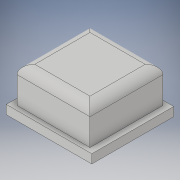
# Autodesk Inventor part: BUTTON2
Saved by Autodesk Inventor 2019 (Build 230136000, 136)
## iProperties
Created: 2018-12-20
Part Number: BUTTON2
Material: Типовые
Document SubType Name: Modeling
Designer: aldanstar
Density: 1 g/cm^3
Appearance: По умолчанию
Author: aldanstar
Autodesk Inventor part; units mm, degrees
ref_plane "YZ Plane" through (0, 0, 0) normal (1, 0, 0) x (0, 1, 0)
ref_plane "XZ Plane" through (0, 0, 0) normal (0, 1, 0) x (-1, 0, 0)
ref_plane "XY Plane" through (0, 0, 0) normal (0, 0, 1) x (1, 0, 0)
sketch "Эскиз1" plane through (0, 0, 0) normal (0, 1, 0) x (-1, 0, 0)
  line L0 (4.1, 4.1) -> (-4.1, 4.1)
  line L1 (-4.1, 4.1) -> (-4.1, -4.1)
  line L2 (-4.1, -4.1) -> (4.1, -4.1)
  line L3 (4.1, -4.1) -> (4.1, 4.1)
  line L4 (5.74, 0) -> (-5.74, 0) projected
  line L5 (0, -5.74) -> (0, 5.74) projected
  point P0 (0, 0)
  dimension "d0" = 8.2
  constraints: 8 end point, 2 parallel, 2 perpendicular, 1 horizontal, 2 other
  measures "d0" distance of L1.end L2.end
extrude "Выдавливание1" add sketch "Эскиз1" along normal blind 5
shell "Оболочка1" thickness 0.8 removed faces 1 at (1.3667, 0, 1.3667)
sketch "Эскиз3" plane through (-3.3, 4.2, 3.3) normal (0, -1, 0) x (1, 0, 0)
  line L0 (0, 0) -> (6.6, 0) projected
  line L1 (6.6, -6.6) -> (0, -6.6) projected
  line L2 (6.6, 0) -> (0, 0)
  line L3 (0, 0) -> (0, -6.6)
  line L4 (0, -6.6) -> (6.6, -6.6)
  line L5 (6.6, -6.6) -> (6.6, 0)
  point P0 (3.3, -3.3)
  constraints: 8 end point, 2 parallel, 1 horizontal, 1 perpendicular
extrude "Выдавливание2" add sketch "Эскиз3" along normal blind 1
fillet "Сопряжение1" radius 1 4 edges at (0, 5, -4.1) (0, 5, 4.1) (4.1, 5, 0) (-4.1, 5, 0)
sketch "Эскиз5" plane through (0, 0, 0) normal (0, -1, 0) x (1, 0, 0)
  line L0 (-4.1, 4.1) -> (4.1, 4.1) projected
  line L1 (4.1, 4.1) -> (4.1, -4.1) projected
  line L2 (4.1, -4.1) -> (-4.1, -4.1) projected
  line L3 (-4.1, -4.1) -> (-4.1, 4.1) projected
  line L4 (-4.6, -4.6) -> (4.6, -4.6)
  line L5 (4.6, -4.6) -> (4.6, 4.6)
  line L6 (4.6, 4.6) -> (-4.6, 4.6)
  line L7 (-4.6, 4.6) -> (-4.6, -4.6)
  line L8 (4.6, -4.6) -> (4.8, -4.6)
  line L9 (4.8, -4.6) -> (4.8, 4.6)
  line L10 (4.8, 4.6) -> (4.6, 4.6)
  line L11 (4.6, 4.6) -> (4.6, -4.6)
  line L12 (-4.6, -4.6) -> (-4.8, -4.6)
  line L13 (-4.8, -4.6) -> (-4.8, 4.6)
  line L14 (-4.8, 4.6) -> (-4.6, 4.6)
  line L15 (-4.6, 4.6) -> (-4.6, -4.6)
  point P0 (0, 0)
  dimension "d10" = 0.5
  dimension "d13" = 0.2
  dimension "d14" = 0.2
  constraints: 24 end point, 4 parallel, 2 horizontal, 2 perpendicular, 3 other
  measures "d10" distance between parallel lines of L4 L2
  measures "d13" distance of L4.end L8.end
  measures "d14" distance of L4.start L12.end
extrude "Выдавливание4" add sketch "Эскиз5" against normal blind 1
chamfer "Фаска1" distance 0.5 angle 45 4 edges at (-3.3, 0, 0) (0, 0, 3.3) (3.3, 0, 0) (0, 0, -3.3)
